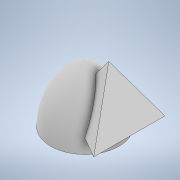
# Autodesk Inventor part: ИДЗ
Saved by Autodesk Inventor 2022 (Build 260153000, 153)
## iProperties
Created: 2023-03-31
Part Number: ИДЗ
Material: Типовые
Document SubType Name: Modeling
Designer: Egor
Density: 1 g/cm^3
Appearance: По умолчанию
Author: Egor
Autodesk Inventor part; units mm, degrees
ref_plane "YZ Plane" through (0, 0, 0) normal (1, 0, 0) x (0, 1, 0)
ref_plane "XY Plane" through (0, 0, 0) normal (0, 0, 1) x (1, 0, 0)
sketch "Эскиз1" plane through (0, 0, 0) normal (0, 1, 0) x (-1, 0, 0)
  line L0 (0, 0) -> (-35, 0)
  circle A0 centre (0, 0) radius 50
  circle A1 centre (-35, 0) radius 60
  line L1 (25, 0) -> (-65, -51.9615)
  line L2 (-65, -51.9615) -> (-65, 51.9615)
  line L3 (-65, 51.9615) -> (25, 0)
  line L4 (-35, 0) -> (-65, -51.9615)
  line L5 (-35, 0) -> (-65, 51.9615)
  line L6 (-35, 0) -> (25, 0)
  dimension "d4" = 120
  dimension "d1" = 35
  dimension "d3" = 100
  constraints: 14 end point, 4 coincident, 1 centre point, 1 collinear, 1 horizontal, 1 horizontal alignment, 9 other
  measures "d1" distance of L0.start L0.end
  measures "d3" diameter of A0
sketch "Эскиз2" plane through (0, 0, 0) normal (0, 1, 0) x (-1, 0, 0)
  line L0 (0, 0) -> (25, 0)
  line L1 (0, 0) -> (-65, 0)
  line L2 (-65, 0) -> (-65, -52)
  line L3 (-65, 0) -> (-65, 52)
  line L4 (-65, 52) -> (25, 0)
  line L5 (25, 0) -> (-65, -52)
  dimension "d5" = 25
  dimension "d6" = 65
  dimension "d7" = 52
  dimension "d8" = 52
  constraints: 12 end point, 2 horizontal, 2 vertical
  measures "d5" distance of L0.start L0.end
  measures "d6" distance of L0.start L1.end
  measures "d7" distance of L1.end L2.end
  measures "d8" distance of L1.end L3.end
ref_plane "РабПлоскость1" through (0, 80, 0) normal (0, 1, 0) x (-1, 0, 0)
sketch "Эскиз3" plane through (0, 80, 0) normal (0, 1, 0) x (-1, 0, 0)
  point P0 (0, 0)
  point P1 (-35, 0)
loft "Лофт1" add profiles "Эскиз2" section 2 point at (35, 80, 0)
sketch "Эскиз7" plane through (0, 0, 0) normal (0, 0, 1) x (1, 0, 0)
  line L0 (0, 0) -> (0, -20)
  line L1 (0, -20) -> (50, -20)
  line L2 (0, -20) -> (-50, -20)
  arc A0 (0, -106.6025) -> (0, 66.6025) centre (-50, -20) ccw
  arc A1 (0, 66.6025) -> (0, -106.6025) centre (50, -20) ccw
  line L3 (0, 0) -> (0, 66.6025)
  dimension "d19" = 20
  dimension "d20" = 50
  dimension "d21" = 50
  dimension "d22" = 200
  dimension "d23" = 200
  constraints: 8 end point, 4 point on circle, 2 centre point, 2 coincident, 1 horizontal, 1 perpendicular, 1 vertical
  measures "d19" distance of L0.start L0.end
  measures "d20" distance of L0.end L1.end
  measures "d21" distance of L0.end L2.end
  measures "d22" diameter of A0
  measures "d23" diameter of A1
revolve "Вращение1" add sketch "Эскиз7" angle 360 about axis through (0, 0, 0) along (0, 1, 0) contours L0 L2 A1 L3
